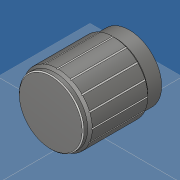
# Autodesk Inventor part: knob
Saved by Autodesk Inventor 2019 (Build 230136000, 136)
## iProperties
Created: 2019-01-06
Part Number: knob
Material: Aluminium 6061
Document SubType Name: Modeling
Designer: Stefan
Mass: 7.05598 g
Surface Area: 13.1203 cm^2
Volume: 2.61333 cm^3
Density: 2.7 g/cm^3
Appearance: Eloxiert - Hellgrau
Author: Stefan
Autodesk Inventor part; units mm, degrees
ref_plane "YZ Plane" through (0, 0, 0) normal (1, 0, 0) x (0, 1, 0)
ref_plane "XZ Plane" through (0, 0, 0) normal (0, 1, 0) x (-1, 0, 0)
ref_plane "XY Plane" through (0, 0, 0) normal (0, 0, 1) x (1, 0, 0)
sketch "Skizze1" plane through (0, 0, 0) normal (0, 0, 1) x (1, 0, 0)
  circle A0 centre (0, 0) radius 7.5
  circle A1 centre (0, 0) radius 7
  circle A2 centre (0, 0) radius 3
  arc A3 (-0.15, -7.4985) -> (0.15, -7.4985) centre (0, 0) ccw
  arc A4 (0.15, -7.4985) -> (-0.15, -7.4985) centre (0, -7.5635) ccw
  line L0 (0, -10.5888) -> (0, 10.5888) projected
  arc A5 (2.731, -6.9851) -> (3.0081, -6.8703) centre (0, 0) ccw
  arc A6 (3.0081, -6.8703) -> (2.731, -6.9851) centre (2.8944, -6.9877) ccw
  arc A7 (5.1962, -5.4083) -> (5.4083, -5.1962) centre (0, 0) ccw
  arc A8 (5.4083, -5.1962) -> (5.1962, -5.4083) centre (5.3482, -5.3482) ccw
  arc A9 (6.8703, -3.0081) -> (6.9851, -2.731) centre (0, 0) ccw
  arc A10 (6.9851, -2.731) -> (6.8703, -3.0081) centre (6.9877, -2.8944) ccw
  arc A11 (7.4985, -0.15) -> (7.4985, 0.15) centre (0, 0) ccw
  arc A12 (7.4985, 0.15) -> (7.4985, -0.15) centre (7.5635, 0) ccw
  arc A13 (6.9851, 2.731) -> (6.8703, 3.0081) centre (0, 0) ccw
  arc A14 (6.8703, 3.0081) -> (6.9851, 2.731) centre (6.9877, 2.8944) ccw
  arc A15 (5.4083, 5.1962) -> (5.1962, 5.4083) centre (0, 0) ccw
  arc A16 (5.1962, 5.4083) -> (5.4083, 5.1962) centre (5.3482, 5.3482) ccw
  arc A17 (3.0081, 6.8703) -> (2.731, 6.9851) centre (0, 0) ccw
  arc A18 (2.731, 6.9851) -> (3.0081, 6.8703) centre (2.8944, 6.9877) ccw
  arc A19 (0.15, 7.4985) -> (-0.15, 7.4985) centre (0, 0) ccw
  arc A20 (-0.15, 7.4985) -> (0.15, 7.4985) centre (0, 7.5635) ccw
  arc A21 (-2.731, 6.9851) -> (-3.0081, 6.8703) centre (0, 0) ccw
  arc A22 (-3.0081, 6.8703) -> (-2.731, 6.9851) centre (-2.8944, 6.9877) ccw
  arc A23 (-5.1962, 5.4083) -> (-5.4083, 5.1962) centre (0, 0) ccw
  arc A24 (-5.4083, 5.1962) -> (-5.1962, 5.4083) centre (-5.3482, 5.3482) ccw
  arc A25 (-6.8703, 3.0081) -> (-6.9851, 2.731) centre (0, 0) ccw
  arc A26 (-6.9851, 2.731) -> (-6.8703, 3.0081) centre (-6.9877, 2.8944) ccw
  arc A27 (-7.4985, 0.15) -> (-7.4985, -0.15) centre (0, 0) ccw
  arc A28 (-7.4985, -0.15) -> (-7.4985, 0.15) centre (-7.5635, 0) ccw
  arc A29 (-6.9851, -2.731) -> (-6.8703, -3.0081) centre (0, 0) ccw
  arc A30 (-6.8703, -3.0081) -> (-6.9851, -2.731) centre (-6.9877, -2.8944) ccw
  arc A31 (-5.4083, -5.1962) -> (-5.1962, -5.4083) centre (0, 0) ccw
  arc A32 (-5.1962, -5.4083) -> (-5.4083, -5.1962) centre (-5.3482, -5.3482) ccw
  arc A33 (-3.0081, -6.8703) -> (-2.731, -6.9851) centre (0, 0) ccw
  arc A34 (-2.731, -6.9851) -> (-3.0081, -6.8703) centre (-2.8944, -6.9877) ccw
  dimension "d0" = 15
  dimension "d3" = 14
  dimension "d14" = 6
  dimension "d20" = 0.3
  dimension "d21" = 0.1
  dimension "d24" = 360
  constraints: 66 point on circle, 35 centre point, 3 coincident, 1 concentric, 1 point on line, 97 other
  measures "d0" diameter of A0
  measures "d3" diameter of A1
  measures "d14" diameter of A2
  measures "d20" distance of A0.start A0.end
extrude "Extrusion1" add sketch "Skizze1" along normal mid plane 17 contours L0 A2 A1 | A1 L0 A2 | L0 A2 | A2 L0
extrude "Extrusion2" add sketch "Skizze1" along normal blind 7 and the other way blind 5 contours A12 A0 A10 A8 A6 A4 L0 A1 A20 A18 A16 A14 | L0 A1 A4 A0 A34 A32 A30 A28 A26 A24 A22 A20
chamfer "Fase1" distance 0.5 angle 45 2 edges at (-7, 0, 7) (-7, 0, -5)
chamfer "Fase2" distance 0.2 angle 45 1 edges at (-7, 0, 8.5)
extrude "Extrusion3" cut sketch "Skizze1" along normal blind 1.5 and the other way blind 8.5 contours L0 A2 | A2 L0
